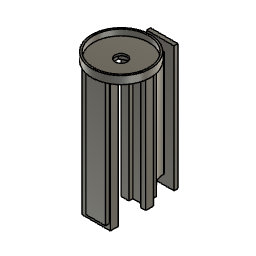
Piston Hood 2 R (Autodesk Fusion 360 design; units mm, degrees)
Autodesk Fusion 360 part; units mm, degrees
sketch "Sketch1" plane through (0, 0, 0) normal (0, 0, 1) x (1, 0, 0) in component "Component"
  circle A0 centre (0, 0) radius 6.5
  line L0 (-3.889087, -2.474874) -> (-5.248582, -3.834369)
  line L1 (0, -2.5) -> (2.165063, -1.25)
  line L2 (0, 2.5) -> (-2.165063, 1.25)
  line L3 (1.732051, 1) -> (0, 2)
  line L4 (3.181981, -3.181981) -> (3.889087, -2.474874)
  line L5 (-1.732051, -1) -> (0, -2)
  line L6 (-2.165063, -1.25) -> (0, -2.5)
  line L7 (3.181981, -3.181981) -> (2.474874, -3.889087)
  line L8 (2.165063, -1.25) -> (2.165063, 1.25)
  circle A1 centre (0, 0) radius 2.75
  line L9 (-3.181981, -3.181981) -> (-2.474874, -3.889087)
  line L10 (0, 2) -> (-1.732051, 1)
  circle A2 centre (0, 0) radius 7.05
  line L11 (3.889087, -2.474874) -> (5.248582, -3.834369)
  line L12 (-3.889087, 2.474874) -> (-5.248582, 3.834369)
  line L13 (-2.165063, 1.25) -> (-2.165063, -1.25)
  circle A3 centre (0, 0) radius 7.5
  line L14 (3.181981, 3.181981) -> (2.474874, 3.889087)
  circle A4 centre (0, 0) radius 1.55
  line L15 (2.474874, -3.889087) -> (3.834369, -5.248582)
  line L16 (-3.181981, 3.181981) -> (-2.474874, 3.889087)
  line L17 (-3.181981, -3.181981) -> (-3.889087, -2.474874)
  line L18 (-2.474874, 3.889087) -> (-3.834369, 5.248582)
  line L19 (3.181981, 3.181981) -> (3.889087, 2.474874)
  line L20 (1.732051, -1) -> (1.732051, 1)
  line L21 (0, -2) -> (1.732051, -1)
  line L22 (3.889087, 2.474874) -> (5.248582, 3.834369)
  line L23 (-2.474874, -3.889087) -> (-3.834369, -5.248582)
  line L24 (-3.181981, 3.181981) -> (-3.889087, 2.474874)
  line L25 (-1.732051, 1) -> (-1.732051, -1)
  line L26 (2.474874, 3.889087) -> (3.834369, 5.248582)
  line L27 (2.165063, 1.25) -> (0, 2.5)
  line L28 (-1.5, -3.5) -> (-2.5, -3.5)
  line L29 (-1.5, -3.5) -> (-1.5, -4.5)
  line L30 (-2.5, -3.5) -> (-3.5, -3.5)
  line L31 (-3.5, -3.5) -> (-3.5, -4.5)
  line L32 (-4.5, -4.5) -> (-3.5, -4.5)
  line L33 (-4.5, -5.5) -> (-4.5, -4.5)
  line L34 (4.5, -5.5) -> (-4.5, -5.5)
  line L35 (4.5, -4.5) -> (4.5, -5.5)
  line L36 (3.5, -4.5) -> (4.5, -4.5)
  line L37 (3.5, -3.5) -> (3.5, -4.5)
  line L38 (2.5, -3.5) -> (3.5, -3.5)
  line L39 (1.5, -3.5) -> (1.5, -4.5)
  line L40 (-1.5, -4.5) -> (1.5, -4.5)
  line L41 (2.5, -3.5) -> (1.5, -3.5)
  line L42 (2.5, 3.5) -> (3.5, 3.5)
  line L43 (3.5, 3.5) -> (3.5, 4.5)
  line L44 (4.5, 4.5) -> (3.5, 4.5)
  line L45 (4.5, 5.5) -> (4.5, 4.5)
  line L46 (-4.5, 5.5) -> (4.5, 5.5)
  line L47 (1.5, 3.5) -> (2.5, 3.5)
  line L48 (1.5, 3.5) -> (1.5, 4.5)
  line L49 (1.5, 4.5) -> (-1.5, 4.5)
  line L50 (-1.5, 3.5) -> (-1.5, 4.5)
  line L51 (-2.5, 3.5) -> (-1.5, 3.5)
  line L52 (-3.5, 3.5) -> (-3.5, 4.5)
  line L53 (-2.5, 3.5) -> (-3.5, 3.5)
  line L54 (-3.5, 4.5) -> (-4.5, 4.5)
  line L55 (-4.5, 4.5) -> (-4.5, 5.5)
  line L56 (0, -5.5) -> (-2.5, -5.5)
  line L57 (-2.5, -5.5) -> (-2.5, -6.5)
  line L58 (-2.5, -6.5) -> (2.5, -6.5)
  line L59 (2.5, -6.5) -> (2.5, -5.5)
  line L60 (2.5, 5.5) -> (2.5, 6.5)
  line L61 (2.5, 6.5) -> (-2.5, 6.5)
  line L62 (-2.5, 6.5) -> (-2.5, 5.5)
  line L63 (0, 10) -> (-1, 10)
  line L64 (-1, 10) -> (-1, 6.5)
  line L65 (0, 10) -> (1, 10)
  line L66 (1, 10) -> (1, 6.5)
  line L67 (0, 11) -> (-3.5, 11)
  line L68 (-3.5, 11) -> (-3.5, 10)
  line L69 (-3.5, 10) -> (3.5, 10)
  line L70 (3.5, 10) -> (3.5, 11)
  line L71 (3.5, 11) -> (0, 11)
  dimension "d1" = 15
  dimension "d2" = 14.1
  dimension "d3" = 13
  dimension "d4" = 3.1
  dimension "d5" = 2
  dimension "d6" = 5.5
  dimension "d17" = 1.922616
  dimension "d18" = 2
  dimension "d19" = 4.5
  dimension "d30" = 1
  dimension "d32" = 360
  dimension "d35" = 2.5
  dimension "d36" = 1
  dimension "d37" = 5
  dimension "d39" = 360
  dimension "d40" = 10
  dimension "d41" = 1
  dimension "d42" = 1
  dimension "d43" = 1
  dimension "d44" = 3.5
  dimension "d45" = 1
  dimension "d46" = 7
  dimension "d47" = 1
  constraint coincident A0.centre A1.centre
  constraint concentric A2 A3
  constraint concentric A2 A4
  constraint concentric A1 A4
  constraint perpendicular L28 L29
  constraint perpendicular L39 L41
  constraint midpoint L34 L56.start
  constraint perpendicular L39 L56
  constraint perpendicular L56 L57
  constraint perpendicular L57 L58
  constraint coincident L34 L59.end
  constraint perpendicular L34 L59
  constraint coincident L61 L64.end
  constraint perpendicular L61 L64
  constraint coincident L61 L66.end
  constraint perpendicular L61 L66
  constraint perpendicular L67 L68
  constraint perpendicular L68 L69
  constraint perpendicular L69 L70
  measures "d1" diameter of A3
  measures "d2" diameter of A2
  measures "d3" diameter of A0
  measures "d4" diameter of A4
  measures "d5" distance of L3.end A0.centre
  measures "d6" diameter of A1
  measures "d30" distance of L28.start L28.end
  measures "d35" distance of L56.start L56.end
  measures "d36" distance of L56.end L57.end
  measures "d37" distance of L57.end L58.end
  measures "d40" distance of A0.centre L63.start
  measures "d41" distance of L63.start L63.end
  measures "d42" distance of L63.start L65.end
  measures "d43" distance of L63.start L67.start
  measures "d44" distance of L67.start L67.end
  measures "d45" distance of L67.end L68.end
  measures "d46" distance of L68.end L69.end
  measures "d47" distance of L69.end L70.end
extrude "Extrude1" add sketch "Sketch1" along normal blind 0.5 contours A0 L0 L4 L7 L9 L11 L12 L14 L16 L17 L19 L22 L24 L28 L29 L30 L38 L39 L40 L41 L42 L47 L48 L49 L50 L51 L53 | A0 A2 L35 L45 | A0 L14 L19 L22 L42 L43 L44 L45 | A0 L4 L7 L11 L35 L36 L37 L38 | A0 L14 L26 L42 L43 L44 L45 | A0 A2 L45 L46 | A0 A2 L34 L35 | A0 L7 L15 L35 L36 L37 L38 | A0 L14 L16 L18 L26 L42 L46 L47 L48 L49 L50 L51 L53 | A2 A3 L33 L34 L35 L45 L46 L55 L64 L66 | A2 L45 L46 | A0 L7 L9 L15 L23 L28 L29 L30 L34 L38 L39 L40 L41 L56 | A2 L34 L35 | A0 L46 L60 | A0 A2 L46 L60 L61 L66 | A0 A2 L34 L57 L58 L59 | A0 L34 L59 | A0 L46 L60 L62 | A0 L60 L61 | A2 L61 L64 L66 | A2 A3 L64 L66 | A0 L58 L59 | A0 L34 L56 L57 L59 | A2 L33 L34 | A0 A2 L33 L34 | A0 L61 L62 | A0 L46 L62 | A0 A2 L46 L61 L62 L64 | A0 L57 L58 | A0 A2 L33 L55 | A0 L34 L57 | A0 A2 L46 L55 | A2 L46 L55 | A0 L9 L23 L30 L31 L32 L33 | A0 L0 L9 L17 L30 L31 L32 L33 | A0 L16 L18 L52 L53 L54 L55 | A0 L12 L16 L24 L52 L53 L54 L55 | L1 L2 L6 L8 L13 L27 | L3 L5 L10 L20 L21 L25 | A1 | A4 picked at (4.35223, 1.234262) picked at (4.747876, -4.943282) picked at (4.212557, 3.269747) picked at (4.212557, -3.269747) picked at (3.287987, 3.833333) picked at (4.283654, 5.128601) picked at (4.283654, -5.128601) picked at (3.287987, -3.833333) picked at (0.5, 5.166667) picked at (-5.027945, -5.135189) picked at (4.470255, 5.475781) picked at (0, -4.833333) picked at (4.470255, -5.475781) picked at (2.610166, 5.783783) picked at (3.091594, 6.11909) picked at (-3.080291, -6.124579) picked at (2.610166, -5.783783) picked at (0, 5.833333) picked at (2.23036, 6.258722) picked at (-0.444779, 6.680689) picked at (-0.778112, 7.151273) picked at (2.23036, -6.258722) picked at (1.397026, -5.758722) picked at (-4.470255, -5.475781) picked at (-4.283654, -5.128601) picked at (-2.23036, 6.258722) picked at (-2.610166, 5.783783) picked at (-3.091594, 6.11909) picked at (-2.23036, -6.258722) picked at (-6.672689, 0) picked at (-2.610166, -5.783783) picked at (-4.283654, 5.128601) picked at (-4.470255, 5.475781) picked at (-3.287987, -3.833333) picked at (-4.212557, -3.269747) picked at (-3.287987, 3.833333) picked at (-4.212557, 3.269747) picked at (-0.721688, -1.916667) picked at (-0.835684, 1.447446) picked at (1.180021, 2.043857) picked at (0.833846, -0.714354)
extrude "Extrude2" add sketch "Sketch1" along normal blind 2 contours A2 A3 L33 L34 L35 L45 L46 L55 L64 L66 | A2 L45 L46 | A2 L34 L35 | A2 A3 L64 L66 | A2 L33 L34 | A2 L46 L55 picked at (-5.027945, -5.135189) picked at (4.470255, 5.475781) picked at (4.470255, -5.475781) picked at (-0.778112, 7.151273) picked at (-4.470255, -5.475781) picked at (-4.470255, 5.475781)
extrude "Extrude3" add sketch "Sketch1" against normal blind 0.5 contours A1 picked at (1.180021, 2.043857)
extrude "Extrude4" cut sketch "Sketch1" along normal blind 1.5 contours A4 picked at (0.833846, -0.714354)
extrude "Extrude5" add sketch "Sketch1" against normal blind 1 contours L1 L2 L6 L8 L13 L27 picked at (-0.721688, -1.916667)
extrude "Extrude6" add sketch "Sketch1" against normal blind 26 contours A0 L14 L26 L42 L43 L44 L45 | A0 A2 L45 L46 | A0 A2 L34 L35 | A0 L7 L15 L35 L36 L37 L38 | A0 L14 L16 L18 L26 L42 L46 L47 L48 L49 L50 L51 L53 | A2 L45 L46 | A0 L7 L9 L15 L23 L28 L29 L30 L34 L38 L39 L40 L41 L56 | A2 L34 L35 | A2 L33 L34 | A0 A2 L33 L34 | A0 A2 L46 L55 | A2 L46 L55 | A0 L9 L23 L30 L31 L32 L33 | A0 L16 L18 L52 L53 L54 L55 picked at (3.287987, 3.833333) picked at (4.283654, 5.128601) picked at (4.283654, -5.128601) picked at (3.287987, -3.833333) picked at (0.5, 5.166667) picked at (4.470255, 5.475781) picked at (0, -4.833333) picked at (4.470255, -5.475781) picked at (-4.470255, -5.475781) picked at (-4.283654, -5.128601) picked at (-4.283654, 5.128601) picked at (-4.470255, 5.475781) picked at (-3.287987, -3.833333) picked at (-3.287987, 3.833333)
extrude "Extrude7" add sketch "Sketch1" against normal blind 24.5 contours A0 L46 L60 L62 | A0 L60 L61 | A0 L61 L62 picked at (0, 5.833333) picked at (2.23036, 6.258722) picked at (-2.23036, 6.258722)
extrude "Extrude8" add sketch "Sketch1" against normal blind 22 contours A2 L61 L64 L66 | A2 A3 L64 L66 | A3 L63 L64 L65 L66 L69 picked at (-0.444779, 6.680689) picked at (-0.778112, 7.151273) picked at (-0.444739, 9.164183)
extrude "Extrude9" cut sketch "Sketch1" against normal blind 2.5 contours A2 L61 L64 L66 | A2 A3 L64 L66 | A3 L63 L64 L65 L66 L69 picked at (-0.444779, 6.680689) picked at (-0.778112, 7.151273) picked at (-0.444739, 9.164183)
extrude "Extrude10" add sketch "Sketch1" against normal blind 24.5 contours L63 L65 L67 L68 L69 L70 L71 picked at (-1.5, 10.666667)
fillet "Fillet1" radius 4.5 2 edges at (1, 6.5, -12.25) (-1, 6.5, -12.25)
extrude "Extrude11" add sketch "Sketch1" against normal blind 24.5 contours A0 L58 L59 | A0 L34 L56 L57 L59 | A0 L57 L58 picked at (2.23036, -6.258722) picked at (1.397026, -5.758722) picked at (-2.23036, -6.258722)
extrude "Extrude12" cut 2 faces at (4.5, 5.166667, -8.666667) (4.5, -4.833333, -8.666667) along direction (-1, 0, 0) blind 1
extrude "Extrude13" cut 2 faces at (3.5, 4.166667, -8.666667) (3.5, -4.166667, -17.333333) along direction (-1, 0, 0) blind 0.75
extrude "Extrude14" add 2 faces at (-1.083333, -5.166667, -26) (-1.083333, 5.166667, -26) along direction (0, 0, -1) blind 7.5
extrude "Extrude15" add 2 faces at (-0.833333, -5.833333, -24.5) (-0.833333, 6.166667, -24.5) along direction (0, 0, -1) blind 7.5
extrude "Extrude16" add 1 faces at (-0.348047, 8.814429, -22) along direction (0, 0, -1) blind 7.5
extrude "Extrude17" add 1 faces at (-0.333333, 10.666667, -24.5) along direction (0, 0, -1) blind 7.5
extrude "Extrude1'" [suppressed] in component "Component"
extrude "Extrude2'" [suppressed] in component "Component"
extrude "Extrude3'" [suppressed] in component "Component"
extrude "Extrude4'" [suppressed] in component "Component"
extrude "Extrude5'" [suppressed] in component "Component"
component "Component" placed x (1, 0, 0) y (0, 1, 0) z (0, 0, 1) at (0, 0, 0)
equation "d33 = -1 mm - 25 mm"
